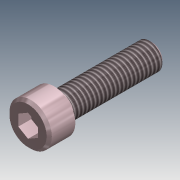
# Autodesk Inventor part: SCREW, SOCKET HD, P, 12.9, M5X0.8X22MM
Saved by Autodesk Inventor 2022.4 (Build 264492000, 492)
## iProperties
Manager: 100-05653
Category: _
Created: 2013-08-06
Material: Generic
Document SubType Name: Modeling
Designer: robr , Rob
Density: 1 g/cm^3
Checked By: 21MJN
Engr Approved By: P
User Status: Released
Description: SCREW, SOCKET HD, P, 12.9, M5X0.8X22MM
Mfg Approved By: Eric.Michaud
Appearance: Glossy - Black
Part Number: SCREW, SOCKET HD, P, 12.9, M5X0.8X22MM
Mass: 0.676013 g
Surface Area: 6.14151 cm^2
Volume: 0.676013 cm^3
Control State: 0
Master: False
Checked Out: False
Shininess: 64.0
CN_SERVICEABLE: _
CN_MASS: 0.000676
CL_runCount: 1
FinishProperty: ToBeSet
FIRST_DESCRIPTION: SCREW, SOCKET HD, P, 12.9, M5X0.8X22MM
SECOND_DESCRIPTION: _
THIRD_DESCRIPTION: _
CN_DETAILER: -
CN_MFG_PART_NUM: FMPSHMA050080022
CN_MFG_NAME: DEFAULT
STANDARDCLASSFLAG: P
CUSTOMERNUMBER: _
CN_DESIGNER: Eric.Michaud
PTC_WM_ITERATION: 4
PTC_WM_ORGANIZATION_ID: CLWC
PTC_WM_LIFECYCLE: CLWC_CAD_LC
Density: 0.0
Volumn: 0.0
Area: 0.0
PropertySet Name: Model Information
Author: -
Revision Number: 1
Subject: FMPSHMA050080022
Keywords: DEFAULT
Autodesk Inventor part; units mm, degrees
ref_plane "YZ Plane" through (0, 0, 0) normal (1, 0, 0) x (0, 1, 0)
ref_plane "XZ Plane" through (0, 0, 0) normal (0, 1, 0) x (-1, 0, 0)
ref_plane "XY Plane" through (0, 0, 0) normal (0, 0, 1) x (1, 0, 0)
sketch "Sketch1" plane through (0, 0, 0) normal (0, 0, 1) x (1, 0, 0)
  circle A0 centre (0, 0) radius 2.5
  dimension "Diameter" = 5
  constraints: 1 centre point
  measures "Diameter" diameter of A0
extrude "Extrusion1" add sketch "Sketch1" along normal blind 22
sketch "Sketch2" plane through (0, 0, 22) normal (0, 0, 1) x (1, 0, 0)
  circle A0 centre (0, 0) radius 2.5 projected
  circle A1 centre (0, 0) radius 4.25
  dimension "Head_Diameter" = 8.5
  constraints: 1 centre point, 1 coincident
  measures "Head_Diameter" diameter of A1
extrude "Extrusion2" add sketch "Sketch2" along normal blind 5 contours A0 | A1
sketch "Sketch3" plane through (0, 0, 27) normal (0, 0, 1) x (1, 0, 0)
  circle A0 centre (0, 0) radius 4.25 projected
  circle A1 centre (0, 0) radius 2.3094 construction
  line L0 (0, 2.3094) -> (2, 1.1547)
  line L1 (2, -1.1547) -> (2, 1.1547)
  line L2 (0, 2.3094) -> (-2, 1.1547)
  line L3 (-2, -1.1547) -> (-2, 1.1547)
  line L4 (-2, -1.1547) -> (0, -2.3094)
  line L5 (2, -1.1547) -> (0, -2.3094)
  dimension "Hex_Width" = 4
  constraints: 12 end point, 6 point on circle, 3 equal length, 1 centre point, 1 coincident, 1 parallel, 1 vertical
  measures "Hex_Width" distance between parallel lines of L0 L4
extrude "Extrusion3" cut sketch "Sketch3" against normal blind 2.5 contours L0 L1 L5 L4 L3 L2
thread "Thread1" size "M5x0.8" class "4g6g" standard "ANSI Metric M Profile" length 22
chamfer "Chamfer1" distance 0.5 angle 45 2 edges at (-4.25, 0, 27) (-2.5, 0, 0)
equation "\"d9\" = ThreadLength"
equation "\"d12\" = Chamfer"
equation "\"ThreadLength\" = 22"
equation "\"Chamfer\" = 0.5"
body "Solid1"
